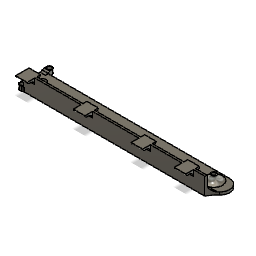
beltPlate (Autodesk Fusion 360 design; units mm, degrees)
Autodesk Fusion 360 part; units mm, degrees
note: some values were not read from the file. Chosen so that the rebuilt part matches the saved one: which pieces of a blend or face edit are solid. Set by a fixed rule: which sketch regions a step uses.
sketch "Sketch1" plane through (0, 0, 0) normal (0, 1, 0) x (1, 0, 0)
  line L0 (0, 0) -> (255, 0)
  line L1 (255, 0) -> (255, -25)
  line L2 (255, -25) -> (0, -25)
  line L3 (0, -25) -> (0, 0)
  line L4 (0, -35) -> (7.1, -35)
  line L5 (7.1, -35) -> (7.1, 10)
  line L6 (7.1, 10) -> (0, 10)
  line L7 (0, 10) -> (0, -35)
  circle A0 centre (3.55, 5) radius 2.55
  circle A1 centre (3.55, -30) radius 2.55
  circle A2 centre (12.15, -12.5) radius 4.75
  dimension "d1" = 255
  dimension "d2" = 25
  dimension "d3" = 7.1
  dimension "d4" = 45
  dimension "d5" = 5.1
  dimension "d6" = 5.1
  dimension "d7" = 35
  dimension "d8" = 9.5
  dimension "d9" = 8.6
  dimension "d10" = 5
  dimension "d11" = 3.55
  dimension "d12" = 3.55
  dimension "d13" = 12.5
  constraint horizontal L0
  constraint vertical L1
  constraint horizontal L2
  constraint vertical L3
  constraint coincident L0.start L3.end
  constraint horizontal L4
  constraint vertical L5
  constraint horizontal L6
  constraint vertical L7
  constraint midpoint L3 L7
  measures "d1" distance of L0.start L0.end
  measures "d2" distance of L0.start L2.end
  measures "d3" distance of L4.start L4.end
  measures "d4" distance of L4.start L6.end
  measures "d5" diameter of A0
  measures "d6" diameter of A1
  measures "d7" vertical distance of A0.centre A1.centre
  measures "d8" diameter of A2
  measures "d9" horizontal distance of A0.centre A2.centre
  measures "d10" distance of L6 A0.centre
  measures "d11" distance of L5 A0.centre
  measures "d12" distance of L5 A1.centre
  measures "d13" distance of L2 A2.centre
extrude "Extrude1" add sketch "Sketch1" along normal blind 3.5
sketch "Sketch2" plane through (0, 3.5, 0) normal (0, 1, 0) x (-1, 0, 0)
  circle A0 centre (-3.55, -5) radius 2.55
  circle A1 centre (-3.55, 30) radius 2.55
  circle A2 centre (-12.15, 12.5) radius 4.75
  line L0 (-7.1, 0) -> (-7.1, -10)
  line L1 (-7.1, -10) -> (0, -10)
  line L2 (0, -10) -> (0, 35)
  line L3 (0, 35) -> (-7.1, 35)
  line L4 (-7.1, 35) -> (-7.1, 25)
  line L5 (-7.1, 25) -> (-255, 25)
  line L6 (-255, 25) -> (-255, 0)
  line L7 (-255, 0) -> (-7.1, 0)
  circle A3 centre (-3.55, 30) radius 3.55
  circle A4 centre (-3.55, -5) radius 3.55
  constraint concentric A1 A3
  constraint tangent L4 A3
  constraint concentric A0 A4
  constraint tangent L0 A4
sketch "Sketch3" plane through (0, 3.5, 0) normal (0, 1, 0) x (-1, 0, 0)
  line L0 (-7.1, 0) -> (-7.1, -10)
  line L1 (-7.1, -10) -> (0, -10)
  line L2 (0, -10) -> (0, 35)
  circle A0 centre (-3.55, -5) radius 2.55
  circle A1 centre (-12.15, 12.5) radius 4.75
  circle A2 centre (-3.55, 30) radius 2.55
  line L3 (0, 35) -> (-7.1, 35)
  line L4 (-7.1, 35) -> (-7.1, 25)
  line L5 (-7.1, 25) -> (-255, 25)
  line L6 (-255, 25) -> (-255, 0)
  line L7 (-255, 0) -> (-7.1, 0)
extrude "Extrude3" cut 1 faces at (4.7333, 1.1667, -10) along direction (0, 0, 1) blind 1.45
extrude "Extrude4" cut 1 faces at (2.3667, 1.1667, 35) along direction (0, 0, -1) blind 1.45
sketch "Sketch4" plane through (0, 3.5, 0) normal (0, 1, 0) x (-1, 0, 0)
  circle A0 centre (-12.15, 12.5) radius 4.75
  line L0 (-7.1, 33.55) -> (-7.1, 25)
  line L1 (-7.1, 25) -> (-255, 25)
  line L2 (-255, 25) -> (-255, 0)
  line L3 (-255, 0) -> (-7.1, 0)
  line L4 (-7.1, 0) -> (-7.1, -8.55)
  line L5 (0, -8.55) -> (0, 33.55)
  circle A1 centre (-234.5, 12.5) radius 2.5
  circle A2 centre (-234.5, 12.5) radius 3.5
  line L6 (0, 33.55) -> (-7.1, 33.55)
  line L7 (-7.1, -8.55) -> (0, -8.55)
  circle A3 centre (-3.55, 30) radius 2.55
  circle A4 centre (-3.55, -5) radius 2.55
  dimension "d24" = 5
  dimension "d25" = 20.5
  dimension "d26" = 12.5
  dimension "d27" = 7
  constraint concentric A1 A2
  measures "d24" diameter of A1
  measures "d25" distance of L2 A1.centre
  measures "d26" distance of L3 A1.centre
  measures "d27" diameter of A2
extrude "Extrude5" add sketch "Sketch4" along normal blind 7.5 contours A1 | A2
fillet "Fillet2" radius 12.5 2 edges at (255, 1.75, 25) (255, 1.75, 0)
sketch "Sketch6" plane through (0, 11, 0) normal (0, 1, 0) x (-1, 0, 0)
  circle A0 centre (-234.5, 12.5) radius 3.5
  circle A1 centre (-234.5, 12.5) radius 2.15
  dimension "d37" = 4.3
  constraint concentric A0 A1
  measures "d37" diameter of A1
extrude "Extrude8" cut sketch "Sketch6" against normal blind 25 contours A1
fillet "Fillet3" radius 7.5 1 edges at (237.7631, 3.5, 13.7657)
extrude "Extrude9" add 1 faces at (164.035, 1.1667, 25) along direction (0, 0, 1) blind 7.5
sketch "Sketch7" plane through (0, 3.5, 0) normal (0, 1, 0) x (-1, 0, 0)
  circle A0 centre (-234.5, 12.5) radius 11
  circle A1 centre (-12.15, 12.5) radius 4.75
  line L0 (-7.1, 32.5) -> (-242.5, 32.5)
  line L1 (-242.5, 32.5) -> (-242.5, 25)
  arc A2 (-242.5, 25) -> (-242.5, 0) centre (-242.5, 12.5) ccw
  line L2 (-242.5, 0) -> (-7.1, 0)
  line L3 (-7.1, 0) -> (-7.1, -8.55)
  line L4 (0, -8.55) -> (0, 33.55)
  line L5 (0, 33.55) -> (-7.1, 33.55)
  line L6 (-7.1, 32.5) -> (-242.5, 32.5)
  line L7 (-242.5, 32.5) -> (-242.5, 30)
  line L8 (-242.5, 30) -> (-7.1, 30)
  line L9 (-7.1, 30) -> (-7.1, 32.5)
  line L10 (-7.1, 33.55) -> (-7.1, 32.5)
  circle A3 centre (-3.55, 30) radius 2.55
  circle A4 centre (-3.55, -5) radius 2.55
  line L11 (-7.1, -8.55) -> (0, -8.55)
  line L12 (-242.5, 32.5) -> (-242.5, 26.1381)
  dimension "d44" = 2.5
  constraint horizontal L6
  constraint vertical L7
  constraint horizontal L8
  constraint vertical L9
  constraint coincident L0.start L6.start
  constraint coincident L0.end L1.start
  constraint coincident L1 L12.end
  constraint perpendicular L0 L12
  constraint collinear L7 L12
  measures "d44" distance of L0.start L8.end
extrude "Extrude10" add sketch "Sketch7" along normal blind 19 contours L0 L1 L6 L7 L8 L9 L12
chamfer "Chamfer1" distance 5 angle 45 1 edges at (124.8, 3.5, 30)
fillet "Fillet4" radius 4.5 2 edges at (124.8, 3.5, 25) (124.8, 8.5, 30)
fillet "Fillet5" radius 37.5 1 edges at (242.5, 1.9521, 25)
sketch "Sketch8" plane through (0, 3.5, 0) normal (0, 1, 0) x (-1, 0, 0)
  line L0 (-237.3062, 23.136) -> (-249.4243, 23.136)
  arc A0 (-250.8121, 21.8359) -> (-249.4243, 23.136) centre (-275.7482, 49.8438) ccw
  arc A1 (-250.8121, 21.8359) -> (-242.5, 0) centre (-242.5, 12.5) ccw
  line L1 (-242.5, 0) -> (-7.1, 0)
  line L2 (-7.1, 0) -> (-7.1, -8.55)
  line L3 (-7.1, -8.55) -> (0, -8.55)
  line L4 (0, -8.55) -> (0, 33.55)
  line L5 (0, 33.55) -> (-7.1, 33.55)
  line L6 (-7.1, 33.55) -> (-7.1, 32.5)
  line L7 (-7.1, 32.5) -> (-7.1, 23.136)
  circle A2 centre (-3.55, -5) radius 2.55
  circle A3 centre (-12.15, 12.5) radius 4.75
  circle A4 centre (-3.55, 30) radius 2.55
  line L8 (-7.1, -8.55) -> (0, -8.55)
  line L9 (0, -8.55) -> (0, 0)
  line L10 (0, 0) -> (-7.1, 0)
  line L11 (-7.1, 0) -> (-7.1, -8.55)
  line L12 (-7.1, 33.55) -> (0, 33.55)
  line L13 (0, 33.55) -> (0, 25)
  line L14 (0, 25) -> (-7.1, 25)
  line L15 (-7.1, 25) -> (-7.1, 33.55)
  line L16 (-7.1, 23.136) -> (-231.6938, 23.136)
  arc A5 (-237.3062, 23.136) -> (-231.6938, 23.136) centre (-234.5, 12.5) ccw
  constraint horizontal L8
  constraint vertical L9
  constraint horizontal L10
  constraint vertical L11
  constraint coincident L9.end L10.start
  constraint coincident L2.end L3.start
  constraint horizontal L12
  constraint vertical L13
  constraint horizontal L14
  constraint vertical L15
  constraint coincident L4 L13.end
  constraint coincident L5.end L6.start
extrude "Extrude11" add sketch "Sketch8" along normal blind 2.1 contours L4 L5 L6 L7 L12 L13 L14 L15 | L2 L3 L4 L8 L9 L10 L11
fillet "Fillet6" radius 2 2 edges at (7.1, 2.8, 32.5) (7.1, 2.8, 33.55)
fillet "Fillet7" radius 3 3 edges at (0, 2.8, 33.55) (0, 2.8, -8.55) (7.1, 2.8, -8.55)
fillet "Fillet8" radius 4 4 edges at (3.55, 3.5, 0) (3.55, 5.6, 0) (3.55, 5.6, 25) (3.55, 3.5, 25)
sketch "Sketch9" plane through (0, 0, 32.5) normal (0, 0, 1) x (1, 0, 0)
  line L0 (8.86, 5.6) -> (8.86, 0)
  line L1 (8.86, 0) -> (242.5, 0)
  line L2 (242.5, 0) -> (242.5, 22.5)
  line L3 (242.5, 22.5) -> (7.1, 22.5)
  line L4 (7.1, 22.5) -> (7.1, 5.6)
  line L5 (7.1, 5.6) -> (8.86, 5.6)
  line L6 (7.1, 22.5) -> (22.1, 22.5)
  line L7 (22.1, 22.5) -> (22.1, 20)
  line L8 (22.1, 20) -> (7.1, 20)
  line L9 (7.1, 20) -> (7.1, 22.5)
  line L10 (7.1, 22.5) -> (7.1, 19.2)
  line L11 (157.1, 22.5) -> (172.1, 22.5)
  line L12 (172.1, 22.5) -> (172.1, 20)
  line L13 (172.1, 20) -> (157.1, 20)
  line L14 (157.1, 20) -> (157.1, 22.5)
  line L15 (97.1, 20) -> (82.1, 20)
  line L16 (82.1, 20) -> (82.1, 22.5)
  line L17 (82.1, 22.5) -> (97.1, 22.5)
  line L18 (97.1, 22.5) -> (97.1, 20)
  line L19 (213.0073, 22.5) -> (228.0073, 22.5)
  line L20 (228.0073, 22.5) -> (228.0073, 20)
  line L21 (228.0073, 20) -> (213.0073, 20)
  line L22 (213.0073, 20) -> (213.0073, 22.5)
  dimension "d60" = 15
  dimension "d61" = 2.5
  dimension "d62" = 15
  dimension "d63" = 2.5
  dimension "d64" = 15
  dimension "d65" = 2.5
  dimension "d79" = 15
  dimension "d80" = 2.5
  constraint horizontal L6
  constraint vertical L7
  constraint horizontal L8
  constraint vertical L9
  constraint coincident L3 L4.start
  constraint coincident L3.end L4.start
  constraint coincident L4 L10.end
  constraint perpendicular L3 L10
  constraint collinear L9 L10
  constraint horizontal L11
  constraint vertical L12
  constraint horizontal L13
  constraint vertical L14
  constraint horizontal L17
  constraint vertical L18
  constraint horizontal L15
  constraint vertical L16
  constraint horizontal L19
  constraint vertical L20
  constraint horizontal L21
  constraint vertical L22
  measures "d60" distance of L3.end L6.end
  measures "d61" distance of L3.end L8.end
  measures "d62" distance of L11.start L11.end
  measures "d63" distance of L13.end L11.start
  measures "d64" distance of L16.end L17.end
  measures "d65" distance of L15.end L16.end
  measures "d79" distance of L19.end L19.start
  measures "d80" distance of L21.end L19.start
extrude "Extrude12" add sketch "Sketch9" along normal blind 10 and the other way blind 7.5 contours L3 L4 L6 L7 L8 L9 L10 | L3 L19 L20 L21 L22 | L3 L11 L12 L13 L14 | L3 L15 L16 L17 L18
fillet "Fillet9" radius 5 4 edges at (164.6, 20, 32.5) (89.6, 20, 32.5) (14.6, 20, 32.5) (220.5073, 20, 32.5)
fillet "Fillet10" radius 2.5 4 edges at (164.6, 20, 42.5) (89.6, 20, 42.5) (14.6, 20, 42.5) (220.5073, 20, 42.5)
fillet "Fillet11" radius 3 6 edges at (14.6, 20, 30) (14.6, 20, 25) (89.6, 20, 30) (89.6, 20, 25) (164.6, 20, 30) (164.6, 20, 25)
sketch "Sketch10" plane through (0, 0, 0) normal (0, -1, 0) x (1, 0, 0)
  arc A0 (4.1, -8.55) -> (7.1, -5.55) centre (4.1, -5.55) ccw
  line L0 (7.1, -5.55) -> (7.1, 0)
  line L1 (7.1, 0) -> (242.5, 0)
  arc A1 (242.5, 0) -> (250.8121, 21.8359) centre (242.5, 12.5) ccw
  arc A2 (242.5, 32.5) -> (250.8121, 21.8359) centre (275.7482, 49.8438) ccw
  line L2 (242.5, 32.5) -> (8.86, 32.5)
  arc A3 (7.5093, 33.025) -> (8.86, 32.5) centre (8.86, 34.5) ccw
  arc A4 (7.5093, 33.025) -> (6.1586, 33.55) centre (6.1586, 31.55) ccw
  line L3 (6.1586, 33.55) -> (3, 33.55)
  arc A5 (3, 33.55) -> (0, 30.55) centre (3, 30.55) ccw
  line L4 (0, 30.55) -> (0, -5.55)
  arc A6 (0, -5.55) -> (3, -8.55) centre (3, -5.55) ccw
  line L5 (3, -8.55) -> (4.1, -8.55)
  circle A7 centre (3.55, 30) radius 2.55
  circle A8 centre (12.15, 12.5) radius 4.75
  circle A9 centre (3.55, -5) radius 2.55
  circle A10 centre (234.5, 12.5) radius 2.15
  line L6 (230.4205, 12.4376) -> (232.5143, 8.9358)
  line L7 (232.5143, 8.9358) -> (236.5938, 8.9982)
  line L8 (236.5938, 8.9982) -> (238.5795, 12.5624)
  line L9 (238.5795, 12.5624) -> (236.4857, 16.0642)
  line L10 (236.4857, 16.0642) -> (232.4062, 16.0018)
  line L11 (232.4062, 16.0018) -> (230.4205, 12.4376)
  point P0 (234.5, 12.5)
  dimension "d76" = 4.08
  constraint coincident P0 A10.centre
  measures "d76" distance of L6.start P0
extrude "Extrude13" cut sketch "Sketch10" against normal blind 1.5 contours L6 L7 L8 L9 L10 L11
equation "d9 = 12.1 mm - 3.5 mm"
equation "d11 = ( 7.10 / 2 ) * 1 mm"
equation "d12 = d11"
equation "d13 = d2 / 2"
equation "d25 = ( 5 / 2 ) * 1 mm + 18 mm"
equation "d26 = ( 25 / 2 ) * 1 mm"
equation "d76 = ( 7.86 mm + 0.3 mm ) / 2"
named bodies: "beltBracket"
